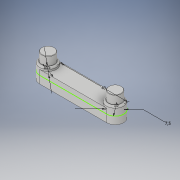
# Autodesk Inventor part: 2er-Stecker
Saved by Autodesk Inventor 2019.5 (Build 235369000, 369)
## iProperties
Created: 2021-09-28
Part Number: 2er-Stecker
Material: Generisch
Document SubType Name: Modeling
Designer: mritt
Density: 1 g/cm^3
Appearance: Vorgabe
Author: mritt
Autodesk Inventor part; units mm, degrees
ref_plane "YZ Plane" through (0, 0, 0) normal (1, 0, 0) x (0, 1, 0)
ref_plane "XZ Plane" through (0, 0, 0) normal (0, 1, 0) x (-1, 0, 0)
ref_plane "XY Plane" through (0, 0, 0) normal (0, 0, 1) x (1, 0, 0)
sketch "Skizze1" plane through (0, 0, 0) normal (0, 1, 0) x (-1, 0, 0)
  line L0 (96.8973, -70.154) -> (56.8973, -70.154)
  circle A0 centre (56.8973, -70.154) radius 5
  circle A1 centre (96.8973, -70.154) radius 5
  circle A2 centre (96.8973, -70.154) radius 3.75
  circle A3 centre (56.8973, -70.154) radius 3.75
  line L1 (96.8973, -65.154) -> (56.8973, -65.154)
  line L2 (56.8973, -65.154) -> (56.8973, -75.154)
  line L3 (56.8973, -75.154) -> (96.8973, -75.154)
  line L4 (96.8973, -75.154) -> (96.8973, -65.154)
  dimension "d8" = 10
  dimension "d11" = 10
  dimension "d12" = 7.5
  dimension "d15" = 7.5
  dimension "d18" = 40
  constraints: 10 end point, 4 centre point, 4 coincident, 2 horizontal, 2 parallel, 1 perpendicular
  measures "d8" diameter of A1
  measures "d11" diameter of A0
  measures "d12" diameter of A2
  measures "d15" diameter of A3
  measures "d18" distance of L2.end L3.end
extrude "Extrusion1" add sketch "Skizze1" along normal blind 10 contours A3 L2 L0 | L0 L2 A3 | L2 A3 | A2 L4 L0 | L0 L4 A2 | L4 A2
extrude "Extrusion2" add sketch "Skizze1" along normal blind 5 contours A0 L2 A3 L0 | L0 A3 L2 A0 | A1 L4 A2 L0 | L0 A2 L4 A1 | L2 A3 A0 | A1 L4 A2
extrude "Extrusion3" add sketch "Skizze1" along normal blind 3 and the other way blind 4.5 contours A0 L2 A3 L0 | A0 L1 A1 L0 | L0 A3 L2 A0 | L0 A1 L3 A0 | A3 L2 L0 | L0 L2 A3 | A1 L4 A2 L0 | L0 A2 L4 A1 | A2 L4 L0 | L0 L4 A2
fillet "Rundung1" radius 1 2 edges at (-51.8973, 5, -70.154) (-91.8973, 5, -70.154)
fillet "Rundung2" radius 0.2 2 edges at (-53.1473, 10, -70.154) (-93.1473, 10, -70.154)
extrude "Extrusion4" add sketch "Skizze1" against normal blind 4.5 contours A0 L2 A3 L0 | L0 A3 L2 A0 | A3 L2 L0 | L0 L2 A3 | A1 L4 A2 L0 | L0 A2 L4 A1 | L2 A3 A0 | L2 A3 | A2 L4 L0 | L0 L4 A2 | A1 L4 A2 | L4 A2
